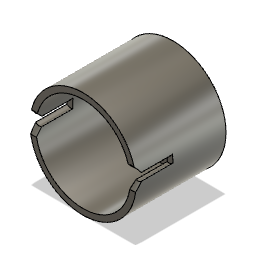
1stSleeve_46mm (Autodesk Fusion 360 design; units mm, degrees)
Autodesk Fusion 360 part; units mm, degrees
sketch "Sketch1" plane through (0, 0, 0) normal (0, 0, 1) x (1, 0, 0)
  circle A0 centre (0, 0) radius 20.5
  circle A1 centre (0, 0) radius 23
  circle A2 centre (0, 0) radius 17.5
  dimension "d1" = 41
  dimension "d2" = 46
  dimension "d30" = 35
  constraint coincident A0.centre A1.centre
  constraint concentric A0 A1
  constraint concentric A1 A2
  measures "d1" diameter of A0
  measures "d2" diameter of A1
  measures "d30" diameter of A2
extrude "Extrude4" add sketch "Sketch1" along normal blind 5 contours A0 makes body 1
extrude "Extrude1" add sketch "Sketch1" along normal blind 39 separate body contours A0 | A1 | A2 makes body 2
extrude "Extrude2" add sketch "Sketch1" along normal blind 8 contours A1 bodies 2
hole "Hole1" at (21.2528, 1.5236, 39) direction (0, 0, -1) diameter 4.5 depth 16 tip angle 180 countersink diameter 9.4 countersink angle 90 bodies 2
hole "Hole2" at (-21.3818, 0.7964, 39) direction (0, 0, -1) diameter 4.5 depth 16 tip angle 180 countersink diameter 9.4 countersink angle 90 bodies 2
hole "Hole3" at (0.0732, 7.1253, 39) direction (0, 0, -1) diameter 4.5 depth 16 tip angle 180 countersink diameter 9.4 countersink angle 90 bodies 2
hole "Hole4" at (0.0701, -8.2193, 39) direction (0, 0, -1) diameter 4.5 depth 16 tip angle 180 countersink diameter 9.4 countersink angle 90 bodies 2
extrude "Extrude3" cut sketch "Sketch1" along normal blind 60 contours A0 | A2 bodies 2
